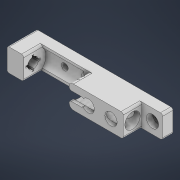
# Autodesk Inventor part: syringe tips fixture
Saved by Autodesk Inventor 2022 (Build 260153000, 153)
## iProperties
Created: 2023-04-13
Part Number: syringe tips fixture
Material: Generic
Document SubType Name: Modeling
Designer: Jakob Saugbjerg
Density: 1 g/cm^3
Appearance: Default
Author: Jakob Saugbjerg
Autodesk Inventor part; units mm, degrees
ref_plane "YZ Plane" through (0, 0, 0) normal (1, 0, 0) x (0, 1, 0)
ref_plane "XZ Plane" through (0, 0, 0) normal (0, 1, 0) x (-1, 0, 0)
ref_plane "XY Plane" through (0, 0, 0) normal (0, 0, 1) x (1, 0, 0)
sketch "Sketch1" plane through (0, 0, 0) normal (0, 0, 1) x (1, 0, 0)
  line L0 (-33, 5.5) -> (33, 5.5)
  line L1 (33, 5.5) -> (33, -5.5)
  line L2 (33, -5.5) -> (-33, -5.5)
  line L3 (-33, -5.5) -> (-33, 5.5)
  line L4 (-33, 5.5) -> (33, -5.5) construction
  line L5 (33, 5.5) -> (-33, -5.5) construction
  point P0 (0, 0)
  dimension "d0" = 66
  dimension "d1" = 11
  constraints: 12 end point, 2 midpoint, 2 parallel, 1 horizontal, 1 perpendicular
  measures "d0" distance of L1.end L2.end
  measures "d1" distance of L0.end L1.end
extrude "Extrusion1" add sketch "Sketch1" along normal blind 5
sketch "Sketch2" plane through (0, 0, 5) normal (0, 0, 1) x (1, 0, 0)
  line L0 (-33, 5.5) -> (-33, -5.5) projected
  line L1 (-33, -5.5) -> (33, -5.5) projected
  line L2 (-33, 5.5) -> (-25, 5.5)
  line L3 (-25, 5.5) -> (-25, -5.5)
  line L4 (-25, -5.5) -> (-33, -5.5)
  line L5 (-33, -5.5) -> (-33, 5.5)
  line L6 (-25, -5.5) -> (-15, -5.5)
  line L7 (33, 5.5) -> (-33, 5.5) projected
  line L8 (-15, -5.5) -> (33, -5.5)
  line L9 (33, -5.5) -> (33, 5.5)
  line L10 (33, 5.5) -> (-15, 5.5)
  line L11 (-15, 5.5) -> (-15, -5.5)
  point P0 (0, 0)
  point P1 (-15, 5.5)
  dimension "d4" = 8
  dimension "d5" = 10
  constraints: 18 end point, 4 parallel, 2 horizontal, 2 perpendicular, 2 point on line
  measures "d4" distance of L3.end L4.end
  measures "d5" distance of L3.end L6.end
extrude "Extrusion2" add sketch "Sketch2" along normal blind 9 contours L2 L3 L1 L0 | L7 L9 L1 L11
sketch "Sketch3" plane through (33, -5.5, 0) normal (1, 0, 0) x (0, 0, -1)
  circle A0 centre (-9.5, 5.5) radius 3.7
  point P0 (0, 5.5)
  dimension "d8" = 7.4
  constraints: 1 centre point
  measures "d8" diameter of A0
extrude "Extrusion3" cut sketch "Sketch3" against normal blind 50
sketch "Sketch4" plane through (-33, -5.5, 0) normal (-1, 0, 0) x (0, 0, 1)
  circle A0 centre (9.5, 5.5) radius 3.7 projected
  circle A1 centre (9.5, 5.5) radius 2.6
  line L0 (9.025, 8.9) -> (9.975, 8.9)
  line L1 (9.975, 8.9) -> (9.975, 2.1)
  line L2 (9.975, 2.1) -> (9.025, 2.1)
  line L3 (9.025, 2.1) -> (9.025, 8.9)
  line L4 (9.025, 8.9) -> (9.975, 2.1) construction
  line L5 (9.975, 8.9) -> (9.025, 2.1) construction
  line L6 (6.1, 5.975) -> (12.9, 5.975)
  line L7 (12.9, 5.975) -> (12.9, 5.025)
  line L8 (12.9, 5.025) -> (6.1, 5.025)
  line L9 (6.1, 5.025) -> (6.1, 5.975)
  line L10 (6.1, 5.975) -> (12.9, 5.025) construction
  line L11 (12.9, 5.975) -> (6.1, 5.025) construction
  point P0 (0, 5.5)
  point P1 (6.9438, 5.975)
  point P2 (6.9438, 5.025)
  point P3 (9.025, 2.9438)
  point P4 (9.975, 2.9438)
  point P5 (9.975, 8.0562)
  point P6 (9.025, 8.0562)
  point P7 (12.0562, 5.975)
  point P8 (12.0562, 5.025)
  dimension "d11" = 5.2
  dimension "d12" = 0.95
  dimension "d13" = 6.8
  dimension "d14" = 6.8
  dimension "d15" = 0.95
  constraints: 24 end point, 4 midpoint, 4 parallel, 2 horizontal, 2 perpendicular, 1 centre point, 1 coincident
  measures "d11" diameter of A1
  measures "d12" distance of L1.end L2.end
  measures "d13" distance of L0.end L1.end
  measures "d14" distance of L7.end L8.end
  measures "d15" distance of L6.end L7.end
extrude "Extrusion4" cut sketch "Sketch4" against normal blind 15 contours A1 L8 L1 L6 | A1 L6 L7 L8 | L6 L1 A1 | A1 L1 L8 | L1 L6 L3 A1 | A1 L3 L0 L1 | L1 L8 L3 L6 | L1 L2 L3 A1 | A1 L3 L8 L1 | L3 L6 A1 | L3 L8 A1 L6 | A1 L8 L3 | A1 L8 L9 L6
sketch "Sketch5" plane through (0, 0, 14) normal (0, 0, 1) x (1, 0, 0)
  line L0 (-15, -3.7) -> (-15, 3.7) projected
  line L1 (-15, 0) -> (-8, 0)
  line L2 (-8, 0) -> (-8, -2.2)
  line L3 (-8, -2.2) -> (-15, -2.2)
  line L4 (-15, -2.2) -> (-15, 0)
  line L5 (-15, 5.5) -> (-15, -5.5) projected
  line L6 (-8, -2.2) -> (-15, -2.2)
  line L7 (-15, -2.2) -> (-15, 2.2)
  line L8 (-15, 2.2) -> (-8, 2.2)
  line L9 (-8, 2.2) -> (-8, -2.2)
  point P0 (0, 0)
  dimension "d18" = 7
  dimension "d19" = 2.2
  dimension "d20" = 4.4
  constraints: 16 end point, 4 parallel, 2 horizontal, 2 perpendicular, 1 midpoint, 1 point on line
  measures "d18" distance of L2.end L3.end
  measures "d19" distance of L1.end L2.end
  measures "d20" distance of L6.end L7.end
extrude "Extrusion5" cut sketch "Sketch5" against normal blind 5
fillet "Fillet1" radius 1 4 edges at (-8, 2.2, 13.2374) (-8, -2.2, 13.2374) (-15, -2.2, 13.2374) (-15, 2.2, 13.2374)
sketch "Sketch6" plane through (33, -5.5, 0) normal (1, 0, 0) x (0, 0, -1)
  line L0 (-5, 0) -> (-5, 11) projected
  line L1 (-14, 0) -> (-14, 11) projected
  line L2 (-5, 0) -> (-14, 0)
  line L3 (-14, 0) -> (-14, 11)
  line L4 (-14, 11) -> (-5, 11)
  line L5 (-5, 11) -> (-5, 0)
  point P0 (0, 5.5)
  constraints: 8 end point, 2 parallel, 1 horizontal, 1 perpendicular
extrude "Extrusion6" cut sketch "Sketch6" against normal blind 10
fillet "Fillet2" radius 1 10 edges at (-33, -5.5, 7) (-25, -5.5, 9.5) (-33, 5.5, 7) (-25, 5.5, 9.5) (-15, 5.5, 9.5) (-15, -5.5, 9.5) (23, -5.5, 9.5) (23, 5.5, 9.5) (33, -5.5, 2.5) (33, 5.5, 2.5)
sketch "Sketch7" plane through (-25, -4.5, 5) normal (1, 0, 0) x (0, 0, -1)
  circle A0 centre (-4.5, 4.5) radius 3.7 projected
  circle A1 centre (-4.5, 4.5) radius 6.25
  point P0 (5, 4.5)
  dimension "d27" = 12.5
  constraints: 1 centre point, 1 coincident
  measures "d27" diameter of A1
extrude "Extrusion7" cut sketch "Sketch7" along normal blind 20
sketch "Sketch8" plane through (0, 0, 14) normal (0, 0, 1) x (1, 0, 0)
  line L0 (-14, -5.5) -> (22, -5.5) projected
  line L1 (-15, 5.5) -> (-3, 5.5)
  line L2 (-3, 5.5) -> (-3, -5.5)
  line L3 (-3, -5.5) -> (-15, -5.5)
  line L4 (-15, -5.5) -> (-15, 5.5)
  point P0 (0, 0)
  dimension "d30" = 12
  constraints: 8 end point, 2 parallel, 1 horizontal, 1 perpendicular, 1 point on line
  measures "d30" distance of L2.end L3.end
extrude "Extrusion8" cut sketch "Sketch8" against normal blind 9
fillet "Fillet3" radius 2 2 edges at (-3, 5.5, 9.5) (-3, -5.5, 9.5)
sketch "Sketch9" plane through (0, 0, 14) normal (0, 0, 1) x (1, 0, 0)
  line L0 (-10, -2.2) -> (4, -2.2)
  line L1 (4, -2.2) -> (4, 2.2)
  line L2 (4, 2.2) -> (-10, 2.2)
  line L3 (-10, 2.2) -> (-10, -2.2)
  line L4 (-3, 3.5) -> (-3, -3.5) projected
  line L5 (-10, -2.2) -> (4, 2.2) construction
  line L6 (4, -2.2) -> (-10, 2.2) construction
  point P0 (0, 0)
  point P1 (-3, 0)
  point P2 (-3, 2.2)
  point P3 (-3, -2.2)
  dimension "d34" = 14
  dimension "d35" = 4.4
  constraints: 12 end point, 3 midpoint, 2 parallel, 1 horizontal, 1 perpendicular
  measures "d34" distance of L2.end L1.end
  measures "d35" distance of L1.end L0.end
extrude "Extrusion9" cut sketch "Sketch9" against normal blind 3 contours L4 L2 L1 L0
fillet "Fillet4" radius 1 4 edges at (-3, 2.2, 13.2374) (4, -2.2, 13.2374) (-3, -2.2, 13.2374) (4, 2.2, 13.2374)
sketch "Sketch10" plane through (0, 0, 5) normal (0, 0, 1) x (1, 0, 0)
  point P0 (0, 0)
sketch "Sketch11" plane through (33, -4.5, 5) normal (0, 0, 1) x (1, 0, 0)
  line L0 (0, 0) -> (0, 9) projected
  line L1 (0, 4.5) -> (-4.85, 4.5)
  circle A0 centre (-4.85, 4.5) radius 1.625
  line L2 (-4.85, 4.5) -> (-15.85, 4.5)
  line L3 (-15.85, 4.5) -> (-26.85, 4.5)
  line L4 (-26.85, 4.5) -> (-37.85, 4.5)
  line L5 (-37.85, 4.5) -> (-48.85, 4.5)
  circle A1 centre (-48.85, 4.5) radius 1.625
  circle A2 centre (-37.85, 4.5) radius 1.625
  circle A3 centre (-26.85, 4.5) radius 1.625
  circle A4 centre (-15.85, 4.5) radius 1.625
  point P0 (-33, 4.5)
  dimension "d39" = 4.85
  dimension "d40" = 3.25
  dimension "d41" = 11
  dimension "d42" = 11
  dimension "d43" = 11
  dimension "d44" = 11
  dimension "d45" = 3.25
  dimension "d46" = 3.25
  dimension "d47" = 3.25
  dimension "d48" = 3.25
  constraints: 10 end point, 5 centre point, 5 coincident, 3 point on line, 2 horizontal, 1 midpoint
  measures "d39" distance of L1.start L1.end
  measures "d40" diameter of A0
  measures "d41" distance of L2.start L2.end
  measures "d42" distance of L2.end L3.end
  measures "d43" distance of L3.end L4.end
  measures "d44" distance of L4.end L5.end
  measures "d45" diameter of A1
  measures "d46" diameter of A2
  measures "d47" diameter of A3
  measures "d48" diameter of A4
extrude "Extrusion10" cut sketch "Sketch11" along normal mid plane 20
sketch "Sketch12" plane through (33, -4.5, 5) normal (0, 0, 1) x (1, 0, 0)
  circle A0 centre (-4.85, 4.5) radius 1.625 projected
  circle A1 centre (-4.85, 4.5) radius 2.95
  line L0 (-4.85, 4.5) -> (-7.8, 4.5)
  circle A2 centre (-15.85, 4.5) radius 2.95
  circle A3 centre (-26.85, 4.5) radius 2.95
  circle A4 centre (-37.85, 4.5) radius 2.95
  circle A5 centre (-48.85, 4.5) radius 2.95
  point P0 (-33, 4.5)
  point P1 (-18.8, 4.5)
  point P2 (-29.8, 4.5)
  point P3 (-40.8, 4.5)
  point P4 (-51.8, 4.5)
  dimension "d51" = 5.9
  dimension "d54" = 11
  constraints: 6 horizontal, 5 horizontal alignment, 2 end point, 1 coincident, 18 other
  measures "d54" distance of point (-4.85, 4.5) point (-15.85, 4.5)
extrude "Extrusion11" cut sketch "Sketch12" along normal blind 20 and the other way blind 3 contours A0 | A1 | A2 | A3 | A4
body "Solid1"
